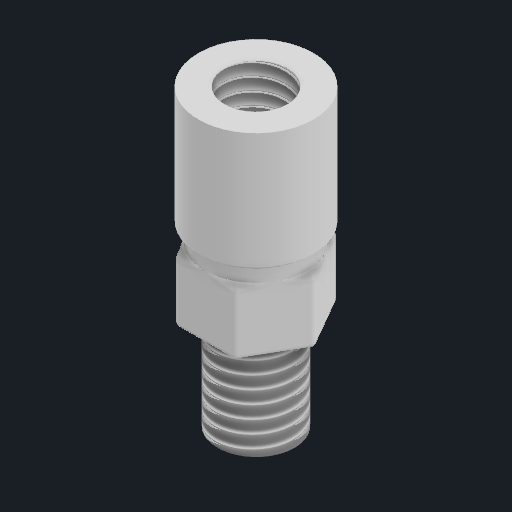
# Autodesk Inventor part: melt zone extender
Saved by Autodesk Inventor 2024.3 (Build 283343000, 343)
## iProperties
Created: 2024-03-20
Part Number: melt zone extender
Material: Generic
Document SubType Name: Modeling
Designer: mateu
Appearance: Default
Surface Area: 9.02349 cm^2
Volume: 0.948869 cm^3
Author: mateu
Autodesk Inventor part; units mm, degrees
ref_plane "YZ Plane" through (0, 0, 0) normal (1, 0, 0) x (0, 1, 0)
ref_plane "XZ Plane" through (0, 0, 0) normal (0, 1, 0) x (-1, 0, 0)
ref_plane "XY Plane" through (0, 0, 0) normal (0, 0, 1) x (1, 0, 0)
sketch "Sketch1" plane through (0, 0, 0) normal (0, 1, 0) x (-1, 0, 0)
  line L0 (-2.309401, -4) -> (-4.618802, 0)
  line L1 (-4.618802, 0) -> (-2.309401, 4)
  line L2 (-2.309401, 4) -> (2.309401, 4)
  line L3 (2.309401, 4) -> (4.618802, 0)
  line L4 (4.618802, 0) -> (2.309401, -4)
  line L5 (2.309401, -4) -> (-2.309401, -4)
  circle A0 centre (0, 0) radius 3
  circle A1 centre (0, 0) radius 1
  dimension "d0" = 8
  dimension "d2" = 6
  dimension "d15" = 2
  constraints: 12 end point, 2 centre point, 2 coincident, 13 other
  measures "d0" distance between parallel lines of L5 L2
  measures "d2" diameter of A0
  measures "d15" diameter of A1
extrude "Extrusion6" add sketch "Sketch1" against normal blind 7.5 contours A0
thread "Thread2" size "M6x1" class "6g" standard "ANSI Metric M Profile" full length
extrude "Extrusion8" add sketch "Sketch1" along normal blind 5 contours L0 L1 L2 L3 L4 L5 | A0
sketch "Sketch4" plane through (0, 5, 0) normal (0, 1, 0) x (1, 0, 0)
  circle A0 centre (0, 0) radius 4
  line L0 (-4.618802, 0) -> (-2.309401, -4)
  line L1 (-2.309401, 4) -> (-4.618802, 0)
  line L2 (-4.618802, 0) -> (-2.309401, -4)
  line L3 (-2.309401, -4) -> (2.309401, -4)
  line L4 (2.309401, -4) -> (4.618802, 0)
  line L5 (4.618802, 0) -> (2.309401, 4)
  line L6 (2.309401, 4) -> (-2.309401, 4)
  circle A1 centre (0, 0) radius 1
  constraints: 1 centre point, 1 coincident, 1 tangent
extrude "Extrusion9" add sketch "Sketch4" along normal blind 1 contours A0
fillet "Fillet2" radius 0.4 24 edges at (4.0415, 5, 1) (2.8868, 5, 3) (1.1547, 5, 4) (4.0415, 5, -1) (2.8868, 5, -3) (1.1547, 5, -4) (-1.1547, 5, -4) (-2.8868, 5, -3) (-4.0415, 5, -1) (-4.0415, 5, 1) (-2.8868, 5, 3) (-1.1547, 5, 4) (2.3094, 2.5, 4) (-2.3094, 2.5, 4) (4.6188, 2.5, 0) (2.3094, 2.5, -4) (-2.3094, 2.5, -4) (-4.6188, 2.5, 0) (-3.4641, 0, -2) (-3.4641, 0, 2) (0, 0, 4) (3.4641, 0, 2) (3.4641, 0, -2) (0, 0, -4)
sketch "Sketch5" plane through (0, 6, 0) normal (0, 1, 0) x (1, 0, 0)
  circle A0 centre (0, 0) radius 4.5
  circle A1 centre (0, 0) radius 4 projected
  circle A2 centre (0, 0) radius 1 projected
  dimension "d49" = 9
  constraints: 1 centre point, 1 coincident
  measures "d49" diameter of A0
extrude "Extrusion10" add sketch "Sketch5" along normal blind 9.5 contours A0 | A1
chamfer "Chamfer3" distance 0.4 angle 45 1 edges at (-4.5, 6, 0)
sketch "Sketch6" plane through (0, 15.5, 0) normal (0, 1, 0) x (1, 0, 0)
  point P0 (0, 0)
  point P1 (0, 0)
  constraints: 1 coincident
hole "Hole3" at (0, 15.5, 0) direction (0, -1, 0) diameter 4.917 depth 7.5 thread size "M6x1" class "6H" standard "ISO Metric profile"
body "Solid2"
